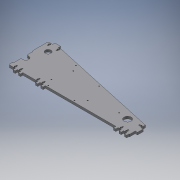
# Autodesk Inventor part: A8-0012
Saved by Autodesk Inventor 2016 SP2 (Build 200236200, 236)
## iProperties
Created: 2017-04-22
Part Number: A8-0012
Material: Generic
Document SubType Name: Modeling
Designer: EV
Density: 1 g/cm^3
Appearance: Default
Author: EV
Autodesk Inventor part; units mm, degrees
ref_plane "YZ Plane" through (0, 0, 0) normal (1, 0, 0) x (0, 1, 0)
sketch "Block1" plane through (0, 0, 0) normal (0, 0, 1) x (1, 0, 0)
  line L0 (-406.7655, -134.7615) -> (-410.2655, -134.7615)
  line L1 (-410.2655, -134.7615) -> (-410.2655, -138.7615)
  line L2 (-410.2655, -138.7615) -> (-411.5155, -138.7615)
  line L3 (-411.5155, -138.7615) -> (-411.5155, -141.7615)
  line L4 (-411.5155, -141.7615) -> (-410.2655, -141.7615)
  line L5 (-410.2655, -141.7615) -> (-410.2655, -146.7615)
  line L6 (-410.2655, -146.7615) -> (-406.7655, -146.7615)
  line L7 (-406.7655, -146.7615) -> (-406.7655, -141.7615)
  line L8 (-406.7655, -141.7615) -> (-405.5155, -141.7615)
  line L9 (-405.5155, -141.7615) -> (-405.5155, -138.7615)
  line L10 (-405.5155, -138.7615) -> (-406.7655, -138.7615)
  line L11 (-406.7655, -138.7615) -> (-406.7655, -134.7615)
  line L12 (-408.5155, -134.7615) -> (-408.5155, -146.7615) construction
  dimension "d28" = 4
  dimension "d29" = 3
  dimension "d30" = 5
  dimension "d31" = 3.5
  dimension "d32" = 6
  measures "d28" distance of L0.end L1.end
  measures "d29" distance of L2.end L3.end
  measures "d30" distance of L4.end L5.end
  measures "d31" distance of L11.end L0.end
  measures "d32" distance between parallel lines of L9 L3
sketch "Sketch1" plane through (0, 0, 0) normal (0, 1, 0) x (-1, 0, 0)
  line L0 (0, 0) -> (0, -12)
  line L1 (0, -12) -> (-3, -15)
  line L2 (0, -137) -> (-15.5, -137)
  line L3 (-15.5, -137) -> (-15.5, -145)
  line L4 (-15.5, -145) -> (-35.5, -145)
  line L5 (-35.5, -145) -> (-35.5, -137)
  line L6 (-35.5, -137) -> (-47.5, -137)
  line L7 (-47.5, -137) -> (-421, -55)
  line L8 (-421, -55) -> (-421, -39.5)
  line L9 (-421, -39.5) -> (-429, -39.5)
  line L10 (-429, -39.5) -> (-429, -19.5)
  line L11 (-429, -19.5) -> (-421, -19.5)
  line L12 (-421, -19.5) -> (-421, 0)
  line L13 (-421, 0) -> (-419, 0)
  line L14 (-419, 0) -> (-419, 8)
  line L15 (-419, 8) -> (-411.5, 8)
  line L16 (-411.5, 8) -> (-411.5, 0)
  line L17 (-411.5, 0) -> (-400, 0)
  line L18 (-400, 0) -> (-400, 8)
  line L19 (-400, 8) -> (-392.5, 8)
  line L20 (-392.5, 8) -> (-392.5, 0)
  line L21 (-392.5, 0) -> (-381, 0)
  line L22 (-381, 0) -> (-381, 8)
  line L23 (-381, 8) -> (-373.5, 8)
  line L24 (-373.5, 8) -> (-373.5, 0)
  line L25 (-373.5, 0) -> (-127.5, 0)
  line L26 (-127.5, 0) -> (-127.5, 8)
  line L27 (-127.5, 8) -> (-120, 8)
  line L28 (-120, 8) -> (-120, 0)
  line L29 (-120, 0) -> (-108.75, 0)
  line L30 (-108.75, 0) -> (-108.75, 8)
  line L31 (-108.75, 8) -> (-101.25, 8)
  line L32 (-101.25, 8) -> (-101.25, 0)
  line L33 (-101.25, 0) -> (-49, 0)
  line L34 (-49, 0) -> (-49, 8)
  line L35 (-49, 8) -> (-41.5, 8)
  line L36 (-41.5, 8) -> (-41.5, 0)
  line L37 (-41.5, 0) -> (-30.25, 0)
  line L38 (-30.25, 0) -> (-30.25, 8)
  line L39 (-30.25, 8) -> (-22.75, 8)
  line L40 (-22.75, 8) -> (-22.75, 0)
  line L41 (-22.75, 0) -> (0, 0)
  line L42 (0, -137) -> (0, -84)
  line L43 (0, -84) -> (-3, -81)
  line L44 (-3, -49.75) -> (-9.75, -49.75) construction
  line L45 (-3, -60) -> (-9.75, -60)
  line L46 (-9.75, -39.5) -> (-3, -39.5)
  arc A0 (-9.75, -39.5) -> (-9.75, -60) centre (-9.75, -49.75) ccw
  line L47 (-3, -81) -> (-3, -60)
  line L48 (-3, -39.5) -> (-3, -15)
  line L49 (-385, 0) -> (-388.5, 0)
  line L50 (-388.5, 0) -> (-388.5, -4)
  line L51 (-388.5, -4) -> (-389.75, -4)
  line L52 (-389.75, -4) -> (-389.75, -7)
  line L53 (-389.75, -7) -> (-388.5, -7)
  line L54 (-388.5, -7) -> (-388.5, -12)
  line L55 (-388.5, -12) -> (-385, -12)
  line L56 (-385, -12) -> (-385, -7)
  line L57 (-385, -7) -> (-383.75, -7)
  line L58 (-383.75, -7) -> (-383.75, -4)
  line L59 (-383.75, -4) -> (-385, -4)
  line L60 (-385, -4) -> (-385, 0)
  line L61 (-386.75, 0) -> (-386.75, -12) construction
  line L62 (-404, 0) -> (-407.5, 0)
  line L63 (-407.5, 0) -> (-407.5, -4)
  line L64 (-407.5, -4) -> (-408.75, -4)
  line L65 (-408.75, -4) -> (-408.75, -7)
  line L66 (-408.75, -7) -> (-407.5, -7)
  line L67 (-407.5, -7) -> (-407.5, -12)
  line L68 (-407.5, -12) -> (-404, -12)
  line L69 (-404, -12) -> (-404, -7)
  line L70 (-404, -7) -> (-402.75, -7)
  line L71 (-402.75, -7) -> (-402.75, -4)
  line L72 (-402.75, -4) -> (-404, -4)
  line L73 (-404, -4) -> (-404, 0)
  line L74 (-405.75, 0) -> (-405.75, -12) construction
  line L75 (-421, -43.5) -> (-421, -47)
  line L76 (-421, -47) -> (-417, -47)
  line L77 (-417, -47) -> (-417, -48.25)
  line L78 (-417, -48.25) -> (-414, -48.25)
  line L79 (-414, -48.25) -> (-414, -47)
  line L80 (-414, -47) -> (-409, -47)
  line L81 (-409, -47) -> (-409, -43.5)
  line L82 (-409, -43.5) -> (-414, -43.5)
  line L83 (-414, -43.5) -> (-414, -42.25)
  line L84 (-414, -42.25) -> (-417, -42.25)
  line L85 (-417, -42.25) -> (-417, -43.5)
  line L86 (-417, -43.5) -> (-421, -43.5)
  line L87 (-421, -45.25) -> (-409, -45.25) construction
  line L88 (-112.625, 0) -> (-116.125, 0)
  line L89 (-116.125, 0) -> (-116.125, -4)
  line L90 (-116.125, -4) -> (-117.375, -4)
  line L91 (-117.375, -4) -> (-117.375, -7)
  line L92 (-117.375, -7) -> (-116.125, -7)
  line L93 (-116.125, -7) -> (-116.125, -12)
  line L94 (-116.125, -12) -> (-112.625, -12)
  line L95 (-112.625, -12) -> (-112.625, -7)
  line L96 (-112.625, -7) -> (-111.375, -7)
  line L97 (-111.375, -7) -> (-111.375, -4)
  line L98 (-111.375, -4) -> (-112.625, -4)
  line L99 (-112.625, -4) -> (-112.625, 0)
  line L100 (-114.375, 0) -> (-114.375, -12) construction
  line L101 (-94.25, 0) -> (-97.75, 0)
  line L102 (-97.75, 0) -> (-97.75, -4)
  line L103 (-97.75, -4) -> (-99, -4)
  line L104 (-99, -4) -> (-99, -7)
  line L105 (-99, -7) -> (-97.75, -7)
  line L106 (-97.75, -7) -> (-97.75, -12)
  line L107 (-97.75, -12) -> (-94.25, -12)
  line L108 (-94.25, -12) -> (-94.25, -7)
  line L109 (-94.25, -7) -> (-93, -7)
  line L110 (-93, -7) -> (-93, -4)
  line L111 (-93, -4) -> (-94.25, -4)
  line L112 (-94.25, -4) -> (-94.25, 0)
  line L113 (-96, 0) -> (-96, -12) construction
  line L114 (-34.125, 0) -> (-37.625, 0)
  line L115 (-37.625, 0) -> (-37.625, -4)
  line L116 (-37.625, -4) -> (-38.875, -4)
  line L117 (-38.875, -4) -> (-38.875, -7)
  line L118 (-38.875, -7) -> (-37.625, -7)
  line L119 (-37.625, -7) -> (-37.625, -12)
  line L120 (-37.625, -12) -> (-34.125, -12)
  line L121 (-34.125, -12) -> (-34.125, -7)
  line L122 (-34.125, -7) -> (-32.875, -7)
  line L123 (-32.875, -7) -> (-32.875, -4)
  line L124 (-32.875, -4) -> (-34.125, -4)
  line L125 (-34.125, -4) -> (-34.125, 0)
  line L126 (-35.875, 0) -> (-35.875, -12) construction
  line L127 (-15.75, 0) -> (-19.25, 0)
  line L128 (-19.25, 0) -> (-19.25, -4)
  line L129 (-19.25, -4) -> (-20.5, -4)
  line L130 (-20.5, -4) -> (-20.5, -7)
  line L131 (-20.5, -7) -> (-19.25, -7)
  line L132 (-19.25, -7) -> (-19.25, -12)
  line L133 (-19.25, -12) -> (-15.75, -12)
  line L134 (-15.75, -12) -> (-15.75, -7)
  line L135 (-15.75, -7) -> (-14.5, -7)
  line L136 (-14.5, -7) -> (-14.5, -4)
  line L137 (-14.5, -4) -> (-15.75, -4)
  line L138 (-15.75, -4) -> (-15.75, 0)
  line L139 (-17.5, 0) -> (-17.5, -12) construction
  line L140 (-11.75, -137) -> (-8.25, -137)
  line L141 (-8.25, -137) -> (-8.25, -133)
  line L142 (-8.25, -133) -> (-7, -133)
  line L143 (-7, -133) -> (-7, -130)
  line L144 (-7, -130) -> (-8.25, -130)
  line L145 (-8.25, -130) -> (-8.25, -125)
  line L146 (-8.25, -125) -> (-11.75, -125)
  line L147 (-11.75, -125) -> (-11.75, -130)
  line L148 (-11.75, -130) -> (-13, -130)
  line L149 (-13, -130) -> (-13, -133)
  line L150 (-13, -133) -> (-11.75, -133)
  line L151 (-11.75, -133) -> (-11.75, -137)
  line L152 (-10, -137) -> (-10, -125) construction
  line L153 (-42.75, -137) -> (-39.25, -137)
  line L154 (-39.25, -137) -> (-39.25, -133)
  line L155 (-39.25, -133) -> (-38, -133)
  line L156 (-38, -133) -> (-38, -130)
  line L157 (-38, -130) -> (-39.25, -130)
  line L158 (-39.25, -130) -> (-39.25, -125)
  line L159 (-39.25, -125) -> (-42.75, -125)
  line L160 (-42.75, -125) -> (-42.75, -130)
  line L161 (-42.75, -130) -> (-44, -130)
  line L162 (-44, -130) -> (-44, -133)
  line L163 (-44, -133) -> (-42.75, -133)
  line L164 (-42.75, -133) -> (-42.75, -137)
  line L165 (-41, -137) -> (-41, -125) construction
  point P0 (-30, -107)
  point P1 (-372, -42)
  point P2 (-132, -5.75)
  point P3 (-223, -5.75)
  point P4 (-119.75, -28.75)
  point P5 (-246, -28.75)
  point P6 (-120, -114)
  point P7 (-223, -92)
  point P8 (-132, -92.75)
  point P9 (-338, -46.75)
  dimension "d0" = 137
  dimension "d2" = 45
  dimension "d3" = 12
  dimension "d4" = 53
  dimension "d5" = 22.75
  dimension "d6" = 7.5
  dimension "d7" = 11.25
  dimension "d8" = 8
  dimension "d9" = 11.25
  dimension "d10" = 11.5
  dimension "d11" = 11.5
  dimension "d12" = 421
  dimension "d13" = 55
  dimension "d14" = 8
  dimension "d15" = 20
  dimension "d16" = 19.5
  dimension "d17" = 101.25
  dimension "d18" = 373.5
  dimension "d19" = 20
  dimension "d20" = 15.5
  dimension "d21" = 8
  dimension "d22" = 47.5
  dimension "d23" = 3
  dimension "d24" = 20.5
  dimension "d26" = 39.5
  dimension "d27" = 17
  dimension "d33" = 4
  dimension "d34" = 3.5
  dimension "d35" = 3.5
  dimension "d36" = 3.75
  dimension "d37" = 3.75
  dimension "d39" = 42
  dimension "d40" = 49
  dimension "d41" = 30
  dimension "d42" = 30
  dimension "d43" = 5.75
  dimension "d44" = 28.75
  dimension "d45" = 46.75
  dimension "d46" = 92
  dimension "d47" = 114
  dimension "d48" = 92.75
  dimension "d49" = 132
  dimension "d50" = 223
  dimension "d51" = 119.75
  dimension "d52" = 246
  dimension "d53" = 338
  dimension "d54" = 132
  dimension "d55" = 223
  dimension "d56" = 120
  constraints: 99 end point, 30 point on line, 26 perpendicular, 16 horizontal, 8 collinear, 6 vertical, 2 horizontal alignment, 2 parallel, 2 point on circle, 2 tangent, 1 centre point
  measures "d0" distance between parallel lines of L2 L41
  measures "d2" angle of L0 L1
  measures "d3" distance of L0.start L0.end
  measures "d4" distance of L2.start L42.end
  measures "d5" distance between parallel lines of L0 L40
  measures "d6" distance of L38.end L39.end
  measures "d7" distance between parallel lines of L36 L38
  measures "d8" distance of L39.end L40.end
  measures "d9" distance between parallel lines of L28 L30
  measures "d10" distance between parallel lines of L20 L22
  measures "d11" distance between parallel lines of L16 L18
  measures "d12" distance between parallel lines of L0 L12
  measures "d13" distance from line of L13 L7.end
  measures "d14" distance of L10.end L11.end
  measures "d15" distance of L9.end L10.end
  measures "d16" distance between parallel lines of L13 L11
  measures "d17" distance between parallel lines of L0 L32
  measures "d18" distance between parallel lines of L0 L24
  measures "d19" distance of L3.end L4.end
  measures "d20" distance between parallel lines of L42 L3
  measures "d21" distance of L2.end L3.end
  measures "d22" distance from line of L6.end L42
  measures "d23" distance between parallel lines of L0 L48
  measures "d24" distance between parallel lines of L45 L46
  measures "d26" distance between parallel lines of L41 L46
  measures "d39" distance from line of point (-372, -42) L25
  measures "d40" distance from line of L12 point (-372, -42)
  measures "d41" distance from line of L42 point (-30, -107)
  measures "d42" distance from line of L2 point (-30, -107)
  measures "d43" distance from line of L25 point (-132, -5.75)
  measures "d44" distance from line of point (-119.75, -28.75) L25
  measures "d45" distance from line of L25 point (-338, -46.75)
  measures "d46" distance from line of L25 point (-223, -92)
  measures "d47" distance from line of L25 point (-120, -114)
  measures "d48" distance from line of L25 point (-132, -92.75)
  measures "d49" distance from line of point (-132, -5.75) L0
  measures "d50" distance from line of point (-223, -5.75) L0
  measures "d51" distance from line of L0 point (-119.75, -28.75)
  measures "d52" distance from line of L0 point (-246, -28.75)
  measures "d53" distance from line of L0 point (-338, -46.75)
  measures "d54" distance from line of L42 point (-132, -92.75)
  measures "d55" distance from line of L42 point (-223, -92)
  measures "d56" distance from line of L42 point (-120, -114)
extrude "Extrusion1" add sketch "Sketch1" along normal blind 8 contours L0 L1 L48 L46 A0 L45 L47 L43 L42 L2 L141 L142 L143 L144 L145 L146 L147 L148 L149 L150 L151 L3 L4 L5 L6 L154 L155 L156 L157 L158 L159 L160 L161 L162 L163 L164 L7 L8 L76 L77 L78 L79 L80 L81 L82 L83 L84 L85 L86 L9 L10 L11 L12 L13 L14 L15 L16 L17 L63 L64 L65 L66 L67 L68 L69 L70 L71 L72 L73 L18 L19 L20 L21 L50 L51 L52 L53 L54 L55 L56 L57 L58 L59 L60 L22 L23 L24 L25 L26 L27 L28 L29 L89 L90 L91 L92 L93 L94 L95 L96 L97 L98 L99 L30 L31 L32 L33 L102 L103 L104 L105 L106 L107 L108 L109 L110 L111 L112 L34 L35 L36 L37 L115 L116 L117 L118 L119 L120 L121 L122 L123 L124 L125 L38 L39 L40 L41 L128 L129 L130 L131 L132 L133 L134 L135 L136 L137 L138
hole "Hole1" at (132, 0, -5.75) at (223, 0, -5.75) at (119.75, 0, -28.75) at (246, 0, -28.75) at (120, 0, -114) at (223, 0, -92) at (132, 0, -92.75) at (338, 0, -46.75) direction (0, 1, 0) diameter 3.5 end through all
hole "Hole2" at (30, 0, -107) direction (0, 1, 0) diameter 20 end through all
hole "Hole3" at (372, 0, -42) direction (0, 1, 0) diameter 25 end through all
fillet "Fillet1" radius 2 8 edges at (0, 4, 0) (0, 4, -12) (3, 4, -15) (3, 4, -81) (0, 4, -84) (0, 4, -137) (3, 4, -60) (3, 4, -39.5)
ref_plane "Work Plane1" through (0, 4, 0) normal (0, 1, 0) x (-1, 0, 0)
ref_plane "Work Plane2" through (405.75, 0, 0) normal (1, 0, 0) x (0, 0, -1)
equation "\"d82\" = 0.5 * THICKNESS"
equation "\"THICKNESS\" = 8"
body "Solid1"
